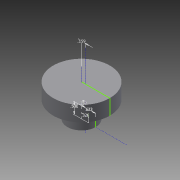
# Autodesk Inventor part: denso-basic
Saved by Autodesk Inventor 2015 (Build 190159000, 159)
## iProperties
Created: 2015-02-04
Part Number: denso-basic
Material: Generic
Document SubType Name: Modeling
Designer: sethbattis
Density: 1 g/cm^3
Appearance: Default
Author: sethbattis
Autodesk Inventor part; units mm, degrees
ref_plane "YZ Plane" through (0, 0, 0) normal (1, 0, 0) x (0, 1, 0)
ref_plane "XZ Plane" through (0, 0, 0) normal (0, 1, 0) x (-1, 0, 0)
ref_plane "XY Plane" through (0, 0, 0) normal (0, 0, 1) x (1, 0, 0)
sketch "Sketch1" plane through (0, 0, 0) normal (0, 0, 1) x (1, 0, 0)
  line L0 (0, 0) -> (0, 50.8) construction
  line L1 (0, 0) -> (50.8, 0) construction
  line L2 (31.75, 18.9992) -> (31.75, 19.1008)
  line L3 (0, 9.5479) -> (15.8115, 9.5479) construction
  line L4 (31.75, 18.9992) -> (15.875, 18.9992)
  line L5 (15.875, 18.9992) -> (15.875, 0)
  line L6 (0, 0) -> (8.2867, 0) construction
  line L7 (8.2867, 0) -> (15.875, 0)
  line L8 (8.2867, 0) -> (8.2867, 12.7)
  line L9 (4.0259, 71.0633) -> (4.0259, -11.3243) construction
  line L10 (8.2867, 12.7) -> (4.0259, 12.7)
  line L11 (4.0259, 19.1008) -> (4.0259, 12.7)
  line L12 (31.75, 36.068) -> (31.75, 19.1008)
  line L13 (31.75, 36.068) -> (0, 36.068)
  line L14 (4.0259, 19.1008) -> (0, 19.1008)
  line L15 (0, 36.068) -> (0, 19.1008)
  dimension "d12" = 15.8115
  dimension "d15" = 8.2867
  dimension "d55" = 4.0259
  dimension "d56" = 12.7
  dimension "d95" = 6.4008
  constraints: 33 end point, 6 point on line, 4 perpendicular, 3 collinear, 3 horizontal, 3 vertical
  measures "d12" distance of L3.start L3.end
  measures "d15" distance of L6.start L6.end
  measures "d55" distance between parallel lines of L0 L9
  measures "d56" distance of L6.end L8.end
  measures "d95" distance of L11.start L10.end
revolve "Revolution1" add sketch "Sketch1" angle 360 about axis through (0, 0, 0) along (0, 1, 0)
sketch "Sketch2" plane through (0, 0, 0) normal (0, -1, 0) x (1, 0, 0)
  circle A0 centre (0, 0) radius 8.2867 construction
  line L0 (-2.2055, 7.9879) -> (-2.2121, 9.8928)
  circle A1 centre (0, 0) radius 10.1371 construction
  line L1 (2.1506, 8.0028) -> (2.144, 9.9078)
  line L2 (-2.2055, 7.9879) -> (2.1506, 8.0028) construction
  arc A2 (2.144, 9.9078) -> (-2.2121, 9.8928) centre (0, 0) ccw
  arc A3 (2.1506, 8.0028) -> (-2.2055, 7.9879) centre (0, 0) ccw
  dimension "d43" = 1.905
  dimension "d44" = 4.3561
  constraints: 8 point on circle, 6 end point, 3 centre point, 2 coincident, 1 concentric, 1 parallel, 1 perpendicular
  measures "d43" distance of L0.start L0.end
  measures "d44" distance of L0.start L1.start
extrude "Extrusion1" cut sketch "Sketch2" against normal blind 12.7
pattern_circular "Circular Pattern2" count 6 over 360 about axis through (0, 6.35, 0) along (0, -1, 0) of "Extrusion1"
body "Solid1"
